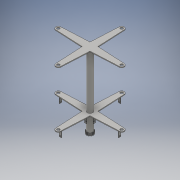
# Autodesk Inventor part: WindCentralbeam
Saved by Autodesk Inventor 2016 SP1 (Build 200210100, 210)
## iProperties
Created: 2016-02-19
Part Number: WindCentralbeam
Material: Generic
Document SubType Name: Modeling
Designer: Tore Den Store
Density: 1 g/cm^3
Appearance: Default
Author: Tore Den Store
Autodesk Inventor part; units mm, degrees
ref_plane "YZ Plane" through (0, 0, 0) normal (1, 0, 0) x (0, 1, 0)
ref_plane "XZ Plane" through (0, 0, 0) normal (0, 1, 0) x (-1, 0, 0)
sketch "Sketch1" plane through (0, 0, 0) normal (0, 0, 1) x (1, 0, 0)
  circle A0 centre (0, 0) radius 100
  dimension "d0" = 200
  constraints: 1 centre point, 1 coincident
  measures "d0" diameter of A0
extrude "Extrusion1" add sketch "Sketch1" along normal blind 2470
ref_plane "End of rigid part plane" through (0, 0, 420) normal (0, 0, 1) x (1, 0, 0)
sketch "Sketch6" plane through (0, 0, 420) normal (0, 0, 1) x (1, 0, 0)
  circle A0 centre (0, 0) radius 100 projected
  circle A1 centre (0, 0) radius 150
  dimension "d56" = 50
  constraints: 1 centre point
  measures "d56" radial gap between concentric circles of A0 A1
extrude "Extrusion7" add sketch "Sketch6" along normal blind 20
sketch "Sketch9" plane through (0, 0, 420) normal (0, 0, -1) x (-1, 0, 0)
  circle A0 centre (0, 0) radius 100 construction
  line L0 (0, 171.6619) -> (0, 152) construction
  line L1 (0, 152) -> (-40, 152)
  line L2 (-40, 152) -> (-40, 162)
  line L3 (-40, 162) -> (40, 162)
  line L4 (40, 162) -> (40, 152)
  line L5 (40, 152) -> (0, 152)
  line L6 (-82.948, 100) -> (83.8994, 100) construction
  circle A1 centre (0, 0) radius 152 construction
  dimension "d122" = 304
  dimension "d77" = 40
  dimension "d78" = 10
  dimension "d79" = 80
  dimension "d123" = 162
  constraints: 14 end point, 3 perpendicular, 2 horizontal, 1 coincident, 1 equal length, 1 tangent, 1 vertical, 3 other
  measures "d77" distance of L0.end L1.end
  measures "d78" distance of L1.end L2.end
  measures "d79" distance of L2.end L3.end
  measures "d123" distance from line of L3 A0.centre
extrude "Extrusion9" add sketch "Sketch9" along normal blind 250
sketch "Sketch14" plane through (-40, 162, 420) normal (0, 1, 0) x (1, 0, 0)
  line L0 (190, 0) -> (-110, 0) projected
  line L1 (40, 0) -> (40, 250) projected
  point P0 (40, 420)
  point P1 (40, 185)
  dimension "d110" = 185
  constraints: 1 point on line
  measures "d110" distance from line of L0 point (40, 185)
hole "Hole4" at (0, 162, 235) direction (0, -1, 0) diameter 40 end up to face face through (13.3333, 152, 336.6667) facing (0, -1, 0)
fillet "Fillet2" radius 2 1 edges at (0, 162, 215)
pattern_circular "Circular Pattern6" count 4 over 360 about axis through (0, 0, 0) along (0, 0, 1) of "Extrusion9", "Hole4", "Fillet2"
sketch "Sketch15" plane through (0, 0, 420) normal (0, 0, 1) x (1, 0, 0)
  circle A0 centre (0, 0) radius 150 projected
  line L0 (40, 162) -> (40, 152) projected
  line L1 (40, 152) -> (40, 144.5683)
  line L2 (40, 162) -> (-40, 162) projected
  line L3 (-40, 162) -> (-40, 152) projected
  line L4 (0, 152) -> (-40, 152) projected
  line L5 (-40, 152) -> (-40, 144.5683)
  constraints: 4 end point, 2 point on circle, 1 collinear, 1 perpendicular
extrude "Extrusion12" add sketch "Sketch15" along normal blind 20 separate body contours A0 L5 L3 L2 L0 L1
pattern_circular "Circular Pattern7" count 4 over 360 about axis through (0, 0, 0) along (0, 0, 1) of "Extrusion12" bodies 2
sketch "Sketch16" plane through (0, 0, 0) normal (0, 0, -1) x (-1, 0, 0)
  circle A0 centre (0, 0) radius 100 projected
extrude "Extrusion13" add sketch "Sketch16" along normal blind 1000 bodies 1
ref_plane "End of rigid" through (0, 0, -130) normal (0, 0, -1) x (-1, 0, 0)
ref_plane "SideOfCylinder" through (0, 100, 0) normal (0, 1, 0) x (-1, 0, 0)
sketch "Sketch17" plane through (0, 100, 0) normal (0, 1, 0) x (-1, 0, 0)
  line L0 (-10, -130) -> (10, -130)
  line L1 (10, -130) -> (10, -230)
  line L2 (10, -230) -> (-10, -230)
  line L3 (-10, -230) -> (-10, -130)
  line L4 (-150, 420) -> (150, 420) projected
  point P0 (0, 0)
  dimension "d133" = 100
  dimension "d135" = 550
  dimension "d136" = 20
  dimension "d138" = 10
  constraints: 8 end point, 2 parallel, 1 horizontal, 1 perpendicular
  measures "d133" distance of L0.end L1.end
  measures "d135" distance between parallel lines of L0 L4
  measures "d136" distance of L0.start L0.end
  measures "d138" distance from line of L1 point (0, 0)
extrude "Extrusion14" add sketch "Sketch17" against normal up to surface round surface about axis through (0, 0, 0) along (0, 0, 1) radius 100 far side no bodies 1
sketch "Sketch18" plane through (0, 100, 0) normal (0, 1, 0) x (1, 0, 0)
  line L0 (0, 130) -> (-10, 130) projected
  line L1 (-10, 130) -> (-10, 230) projected
  line L2 (-10, 230) -> (0, 230) projected
  line L3 (0, 230) -> (10, 230) projected
  line L4 (10, 230) -> (10, 130) projected
  line L5 (10, 130) -> (0, 130) projected
  line L6 (100, 1000) -> (-100, 1000) projected
  line L7 (100, -420) -> (-100, -420) projected
  point P0 (0, 0)
extrude "Extrusion15" add sketch "Sketch18" along normal blind 25 bodies 1
sketch "Sketch19" plane through (0, 0, -130) normal (0, 0, 1) x (1, 0, 0)
  line L0 (10, 125) -> (10, 99.4987) projected
  line L1 (10, 114.4987) -> (6.1779, 125)
  line L2 (10, 125) -> (-10, 125) projected
  line L3 (-6.1779, 125) -> (-10, 114.4987)
  line L4 (10, 114.4987) -> (10, 125)
  line L5 (-10, 125) -> (-10, 99.4987) projected
  line L6 (-6.1779, 125) -> (-10, 125)
  line L7 (-10, 125) -> (-10, 114.4987)
  point P0 (0, 0)
  dimension "d143" = 15
  dimension "d144" = 20
  dimension "d145" = 20
  constraints: 10 end point, 6 point on line, 1 collinear, 1 equal length, 1 horizontal
  measures "d143" distance of L5.end L3.end
  measures "d144" angle of L5 L3
  measures "d145" angle of L1 L0
extrude "Extrusion16" cut sketch "Sketch19" against normal up to surface (100 mm away) bodies 1
pattern_circular "Circular Pattern8" count 16 over 360 about axis through (0, 0, 0) along (0, 0, 1) of "Extrusion14", "Extrusion15", "Extrusion16" bodies 1
sketch "Sketch20" plane through (0, 0, 440) normal (0, 0, 1) x (1, 0, 0)
  circle A0 centre (0, 0) radius 150 construction
  line L0 (0, 0) -> (-141.4214, -141.4214)
  arc A1 (-1154.5723, 89.8838) -> (-1154.5723, -89.8838) centre (-1150, 0) ccw
  line L1 (-1154.5723, 89.8838) -> (-141.4214, 141.4214)
  line L2 (-141.4214, 141.4214) -> (0, 0)
  line L3 (-1154.5723, -89.8838) -> (-141.4214, -141.4214)
  line L4 (-141.4214, -141.4214) -> (-282.8427, 0)
  line L5 (-282.8427, 0) -> (-141.4214, 141.4214)
  line L6 (-282.8427, 0) -> (0, 0)
  dimension "d151" = 90
  dimension "d152" = 200
  dimension "d154" = 1150
  constraints: 14 end point, 3 perpendicular, 2 equal length, 2 point on circle, 2 tangent, 1 centre point, 1 horizontal
  measures "d151" radius of A1
  measures "d152" distance of L1.end L0.start
  measures "d154" distance of point (0, 0) A1.centre
extrude "Extrusion17" add sketch "Sketch20" along normal blind 30 bodies 1
sketch "Sketch21" plane through (0, 0, 470) normal (0, 0, 1) x (1, 0, 0)
  arc A0 (-1154.5723, 89.8838) -> (-1154.5723, -89.8838) centre (-1150, 0) ccw projected
  point P0 (0, 0)
  dimension "d157" = 0
  measures "d157" distance of A0.centre point (-1150, 0)
hole "Hole5" at (-1150, 0, 470) direction (0, 0, -1) diameter 100 end up to face face through (-819.7148, 0, 440) facing (0, 0, -1) bodies 1
pattern_circular "Circular Pattern9" count 4 over 360 about axis through (0, 0, 0) along (0, 0, 1) of "Extrusion17", "Hole5" bodies 1
sketch "Sketch22" plane through (0, 0, 440) normal (0, 0, -1) x (-1, 0, 0)
  line L0 (-1077, -40) -> (-1067, -40)
  line L1 (-1067, -40) -> (-1067, 40)
  line L2 (-1067, 40) -> (-1077, 40)
  line L3 (-1077, 40) -> (-1077, -40)
  circle A0 centre (-1150, 0) radius 50 projected
  line L4 (-162, -40) -> (-162, 40) projected
  point P0 (0, 0)
  dimension "d169" = 40
  dimension "d186" = 10
  dimension "d187" = 80
  dimension "d188" = 905
  constraints: 8 end point, 2 parallel, 1 horizontal, 1 perpendicular
  measures "d169" distance from line of A0.centre L0
  measures "d186" distance of L1.end L2.end
  measures "d187" distance of L2.end L0.start
  measures "d188" distance between parallel lines of L1 L4
extrude "Extrusion18" add sketch "Sketch22" along normal blind 250 contours L3 L2 L1 L0 bodies 1
sketch "Sketch23" plane through (1077, -40, 440) normal (1, 0, 0) x (0, 0, -1)
  line L0 (0, 80) -> (0, 0) projected
  line L1 (0, 0) -> (250, 0) projected
  point P0 (440, 40)
  point P1 (205, 40)
  dimension "d172" = 205
  dimension "d173" = 40
  measures "d172" distance from line of point (205, 40) L0
  measures "d173" distance from line of L1 point (205, 40)
hole "Hole6" at (1077, 0, 235) direction (-1, 0, 0) diameter 40 end up to face face through (1067, 13.3333, 356.6667) facing (-1, 0, 0) bodies 1
fillet "Fillet3" radius 2 1 edges at (1077, 0, 255)
fillet "Fillet4" radius 2 1 edges at (1067, 0, 255)
pattern_circular "Circular Pattern10" count 4 over 360 about axis through (0, 0, 0) along (0, 0, 1) of "Extrusion18", "Hole6", "Fillet3", "Fillet4" bodies 1
sketch "Sketch24" plane through (0, 0, -1000) normal (0, 0, -1) x (-1, 0, 0)
  circle A0 centre (0, 0) radius 100 projected
extrude "Extrusion19" cut sketch "Sketch24" against normal up to surface (770 mm away) bodies 1
ref_plane "Work Plane11" through (0, 0, 1470) normal (0, 0, 1) x (1, 0, 0)
mirror "Mirror3" about plane through (0, 0, 1470) normal (0, 0, 1) of "Extrusion17", "Hole5", "Circular Pattern9" bodies 1
equation "\"d145\" = d144"
body "Solid5"
